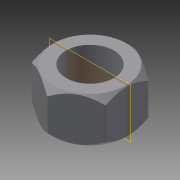
# Autodesk Inventor part: 9mmRodNut
Saved by Autodesk Inventor 2015 (Build 190159000, 159)
## iProperties
Created: 2017-03-08
Part Number: 9mmRodNut
Material: Generic
Document SubType Name: Modeling
Designer: Ernest
Density: 1 g/cm^3
Appearance: Default
Author: Ernest
Autodesk Inventor part; units mm, degrees
ref_plane "YZ Plane" through (0, 0, 0) normal (1, 0, 0) x (0, 1, 0)
ref_plane "XZ Plane" through (0, 0, 0) normal (0, 1, 0) x (-1, 0, 0)
ref_plane "XY Plane" through (0, 0, 0) normal (0, 0, 1) x (1, 0, 0)
sketch "Sketch1" plane through (0, 0, 0) normal (0, 0, 1) x (1, 0, 0)
  circle A0 centre (0, 0) radius 4.5
  line L0 (0, 8.0829) -> (7, 4.0415)
  line L1 (7, 4.0415) -> (7, -4.0415)
  line L2 (7, -4.0415) -> (0, -8.0829)
  line L3 (0, -8.0829) -> (-7, -4.0415)
  line L4 (-7, -4.0415) -> (-7, 4.0415)
  line L5 (-7, 4.0415) -> (0, 8.0829)
  dimension "d0" = 9
  dimension "d1" = 14
  constraints: 12 end point, 2 coincident, 1 centre point, 13 other
  measures "d0" diameter of A0
  measures "d1" distance between parallel lines of L2 L5
extrude "Extrusion1" add sketch "Sketch1" along normal blind 8.4
fillet "Fillet1" radius 0.2 6 edges at (0, 8.0829, 4.2) (7, 4.0415, 4.2) (7, -4.0415, 4.2) (0, -8.0829, 4.2) (-7, -4.0415, 4.2) (-7, 4.0415, 4.2)
ref_plane "Work Plane1" through (14, 0, 0) normal (0, -1, 0) x (0, 0, -1)
sketch "Sketch2" plane through (14, 0, 0) normal (0, -1, 0) x (0, 0, -1)
  line L0 (-8.4, -18.5) -> (-8.4, -9.5) projected
  line L1 (0, -9.5) -> (0, -18.5) projected
  line L2 (-8.4, -21) -> (-8.4, -20.9) projected
  line L3 (-8.4, -20.9) -> (-8.4, -21) projected
  line L4 (-8.4, -20.9) -> (-8.4, -14.1) projected
  line L5 (-8.4, -13.9) -> (-8.4, -14.1) projected
  line L6 (-8.4, -13.9) -> (-8.4, -7.1) projected
  line L7 (-8.4, -7) -> (-8.4, -7.1) projected
  line L8 (-8.4, -7.1) -> (-8.4, -7) projected
  line L9 (-8.4, -7.1) -> (-8.4, -13.9) projected
  line L10 (-8.4, -14.1) -> (-8.4, -13.9) projected
  line L11 (-8.4, -14.1) -> (-8.4, -20.9) projected
  line L12 (-8.4, -18.5) -> (-8.4, -9.5) projected
  line L13 (0, -14) -> (-8.4, -14) construction
  line L14 (-8.4, -18.5) -> (-8.4, -9.5) projected
  line L15 (0, -7) -> (-8.4, -7) projected
  line L16 (-8.4, -7) -> (0, -7) projected
  line L17 (-11.2148, -9.9562) -> (-6.1403, -4.8817)
  line L18 (-6.1403, -4.8817) -> (-8.7846, -2.2375)
  line L19 (-8.7846, -2.2375) -> (-13.859, -7.3119)
  line L20 (-13.859, -7.3119) -> (-11.2148, -9.9562)
  line L21 (-2.4359, -4.7055) -> (1.9907, -9.1321)
  line L22 (1.9907, -9.1321) -> (4.5972, -6.5255)
  line L23 (4.5972, -6.5255) -> (0.1707, -2.099)
  line L24 (0.1707, -2.099) -> (-2.4359, -4.7055)
  dimension "d5" = 45
  dimension "d6" = 0.1
  dimension "d7" = 45
  dimension "d8" = 0.1
  constraints: 18 end point, 6 perpendicular, 2 other
  measures "d5" angle of L16 L17
  measures "d6" distance from line of L7.start L17
  measures "d7" angle of L16 L21
  measures "d8" distance from line of L15.start L21
revolve "Revolution1" cut sketch "Sketch2" angle 360 about axis through (0, 0, 0) along (0, 0, 1)
body "Solid1"
